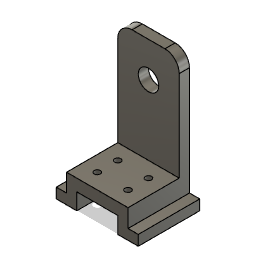
axial+holder (Autodesk Fusion 360 design; units mm, degrees)
Autodesk Fusion 360 part; units mm, degrees
note: some values were not read from the file. Chosen so that the rebuilt part matches the saved one: a direction.
sketch "Sketch1" plane through (0, 0, 0) normal (0, 0, 1) x (1, 0, 0)
  line L0 (85.6912, 5) -> (85.6912, 58)
  line L1 (55.6912, 58) -> (55.6912, 5)
  line L2 (80.6912, 0) -> (80.6912, 8)
  line L3 (80.6912, 8) -> (60.6912, 8)
  line L4 (60.6912, 8) -> (60.6912, 0)
  line L5 (78.6912, 65) -> (62.6912, 65)
  line L6 (50.6912, 0) -> (60.6912, 0)
  circle A0 centre (70.6912, 47.793) radius 5
  line L7 (70.6912, 65) -> (70.6912, 26.651) construction
  line L8 (50.6912, 0) -> (50.6912, 5)
  line L9 (55.6912, 13.8) -> (85.6912, 13.8)
  line L10 (90.6912, 5) -> (90.6912, 0)
  line L11 (90.6912, 0) -> (80.6912, 0)
  line L12 (50.6912, 5) -> (55.6912, 5)
  line L13 (85.6912, 5) -> (90.6912, 5)
  arc A1 (62.6912, 65) -> (55.6912, 58) centre (62.6912, 58) ccw
  arc A2 (85.6912, 58) -> (78.6912, 65) centre (78.6912, 58) ccw
  dimension "d1" = 20
  dimension "d2" = 8
  dimension "d9" = 10
  dimension "d12" = 5.8
  dimension "d13" = 10
  dimension "d14" = 10
  dimension "d15" = 5
  dimension "d16" = 5
  dimension "d17" = 5
  dimension "d18" = 5
  dimension "d19" = 47.793
  dimension "d20" = 65
  dimension "d21" = 7
  constraint horizontal L6
  constraint vertical L0
  constraint vertical L1
  constraint vertical L2
  constraint horizontal L3
  constraint vertical L4
  constraint horizontal L5
  constraint perpendicular L5 L7
  constraint coincident A0.centre L7
  constraint perpendicular L6 L8
  constraint perpendicular L1 L9
  constraint perpendicular L2 L11
  constraint perpendicular L10 L12
  constraint coincident L0.start L12
  constraint collinear L12 L13
  constraint coincident L0 L9.end
  constraint coincident L1 L9.start
  constraint horizontal L13
  constraint coincident L5 L7.start
  constraint tangent L1 A1
  constraint tangent L5 A1
  constraint tangent L5 A2
  constraint tangent L0 A2
  constraint equal A1 A2
  measures "d1" distance of L2 L4
  measures "d2" distance of L3 L6
  measures "d9" diameter of A0
  measures "d12" distance of L3 L9
  measures "d13" distance of L4.end L6.start
  measures "d14" distance of L2.start L10.end
  measures "d15" distance of L10.start L0.start
  measures "d16" horizontal distance of L8.end L1.end
  measures "d17" vertical distance of L10.end L10.start
  measures "d18" distance of L6.start L8.end
  measures "d19" distance of A0.centre L11
  measures "d20" distance of L5 L11
  measures "d21" radius of A1
extrude "Extrude1" add sketch "Sketch1" along normal blind 5 contours L0 L1 L5 L9 A1 A2
extrude "Extrude2" add sketch "Sketch1" along normal blind 30 contours L0 L1 L2 L3 L4 L6 L8 L9 L10 L11 L12 L13
sketch "Sketch2" plane through (0, 13.8, 0) normal (0, 1, 0) x (-1, 0, 0)
  line L0 (-85.6912, 5) -> (-55.6912, 5)
  line L1 (-55.6912, 5) -> (-55.6912, 30)
  line L2 (-55.6912, 30) -> (-85.6912, 30)
  line L3 (-85.6912, 30) -> (-85.6912, 5)
  line L4 (-63.185, 12.5052) -> (-78.185, 12.5052) construction
  line L5 (-78.185, 12.5052) -> (-78.185, 22.5052) construction
  line L6 (-78.185, 22.5052) -> (-63.185, 22.5052) construction
  line L7 (-63.185, 22.5052) -> (-63.185, 12.5052) construction
  line L8 (-70.685, 17.4948) -> (-70.685, 17.5052)
  circle A0 centre (-63.185, 12.5052) radius 1.5
  circle A1 centre (-78.185, 12.5052) radius 1.5
  circle A2 centre (-78.185, 22.5052) radius 1.5
  circle A3 centre (-63.185, 22.5052) radius 1.5
  dimension "d26" = 15
  dimension "d27" = 10
  dimension "d28" = 3
  constraint horizontal L4
  constraint vertical L5
  constraint horizontal L6
  constraint vertical L7
  constraint coincident L4.start L7.end
  constraint coincident L4.end L5.start
  constraint coincident L5.end L6.start
  constraint coincident L6.end L7.start
  constraint equal A0 A1
  constraint equal A1 A3
  constraint equal A2 A3
  measures "d26" distance of L4.start L4.end
  measures "d27" distance of L4.start L6.end
  measures "d28" diameter of A0
extrude "Extrude3" cut sketch "Sketch2" against normal through all contours A0 | A1 | A2 | A3
